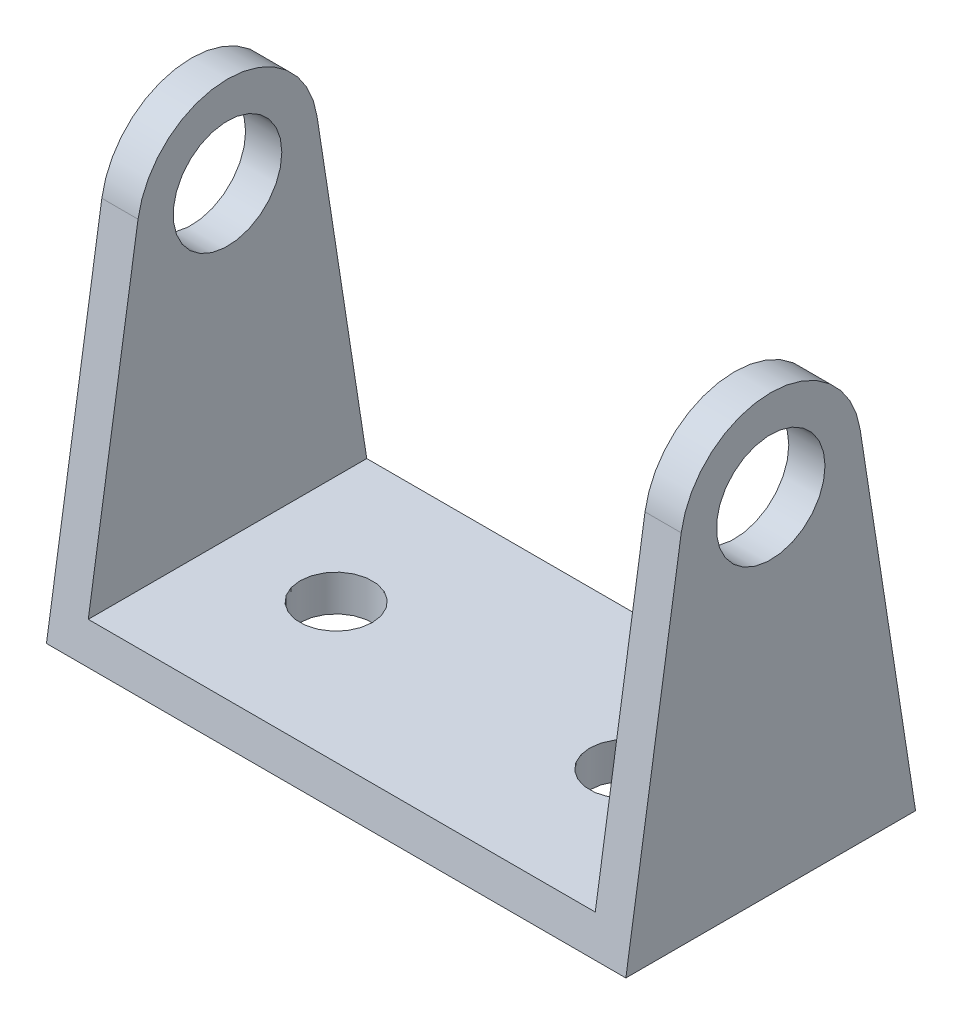
# Autodesk Inventor part: manipulator U bracket
Saved by Autodesk Inventor 2012 (Build 160160000, 160)
## iProperties
Created: 2013-09-01
Part Number: manipulator U bracket
Material: Default
Document SubType Name: Modeling
Designer: Bryce
Density: 1 g/cm^3
Author: Bryce
Autodesk Inventor part; units mm, degrees
ref_plane "YZ Plane" through (0, 0, 0) normal (1, 0, 0) x (0, 1, 0)
ref_plane "XZ Plane" through (0, 0, 0) normal (0, 1, 0) x (-1, 0, 0)
ref_plane "XY Plane" through (0, 0, 0) normal (0, 0, 1) x (1, 0, 0)
sketch "Sketch1" plane through (0, 0, 0) normal (0, 0, 1) x (1, 0, 0)
  line L0 (0, 0) -> (50.8, 0)
  line L1 (50.8, 0) -> (50.8, 38.1)
  line L2 (0, 38.1) -> (0, 0)
  line L3 (3.175, 38.1) -> (3.175, 3.175)
  line L4 (3.175, 3.175) -> (47.625, 3.175)
  line L5 (47.625, 3.175) -> (47.625, 38.1)
  line L6 (50.8, 38.1) -> (47.625, 38.1)
  line L7 (3.175, 38.1) -> (0, 38.1)
  dimension "d0" = 38.1
  dimension "d1" = 50.8
  dimension "d2" = 3.175
  dimension "d3" = 3.175
  dimension "d4" = 3.175
  constraints: 16 end point, 4 parallel, 1 collinear, 1 horizontal, 1 perpendicular
  measures "d0" distance of L2.start L0.start
  measures "d1" distance of L0.start L0.end
  measures "d2" distance between parallel lines of L2 L3
  measures "d3" distance between parallel lines of L0 L4
  measures "d4" distance between parallel lines of L1 L5
extrude "Extrusion1" add sketch "Sketch1" along normal blind 25.4
sketch "Sketch2" plane through (50.8, 0, 0) normal (1, 0, 0) x (0, 0, -1)
  line L0 (-25.4, 38.1) -> (-25.4, 0) projected
  line L1 (0, 0) -> (-25.4, 0) projected
  line L2 (0, 0) -> (0, 38.1) projected
  line L3 (0, 38.1) -> (-25.4, 38.1) projected
  circle A0 centre (-12.7, 30.1625) radius 4.7625
  arc A1 (-4.8559, 31.3765) -> (-20.5441, 31.3765) centre (-12.7, 30.1625) ccw
  line L4 (-25.4, 0) -> (-20.5441, 31.3765)
  line L5 (-4.8559, 31.3765) -> (0, 0)
  dimension "d7" = 9.525
  dimension "d8" = 30.1625
  dimension "d9" = 12.7
  constraints: 4 end point, 3 tangent, 2 centre point, 2 point on circle, 1 coincident
  measures "d7" diameter of A0
  measures "d8" distance from line of L1 A0.centre
  measures "d9" distance from line of L0 A0.centre
extrude "Extrusion2" cut sketch "Sketch2" against normal through all contours L3 A1 L4 L0 | L3 L2 L5 A1 | A0
sketch "Sketch3" plane through (0, 0, 25.4) normal (0, -1, 0) x (1, 0, 0)
  line L0 (0, -25.4) -> (0, 0) projected
  line L1 (0, -25.4) -> (50.8, -25.4) projected
  line L2 (50.8, -25.4) -> (50.8, 0) projected
  circle A0 centre (12.7, -12.7) radius 3.175
  circle A1 centre (38.1, -12.7) radius 3.175
  dimension "d12" = 6.35
  dimension "d13" = 6.35
  dimension "d14" = 12.7
  dimension "d15" = 12.7
  dimension "d16" = 12.7
  constraints: 2 centre point, 1 horizontal alignment
  measures "d12" diameter of A0
  measures "d13" diameter of A1
  measures "d14" distance from line of L1 A0.centre
  measures "d15" distance from line of A0.centre L0
  measures "d16" distance from line of L2 A1.centre
extrude "Extrusion3" cut sketch "Sketch3" against normal through all
equation "\"d3\" = d2"
equation "\"d4\" = d3"
equation "\"d13\" = d12"
equation "\"d15\" = d14"
equation "\"d16\" = d15"
body "Solid1"
